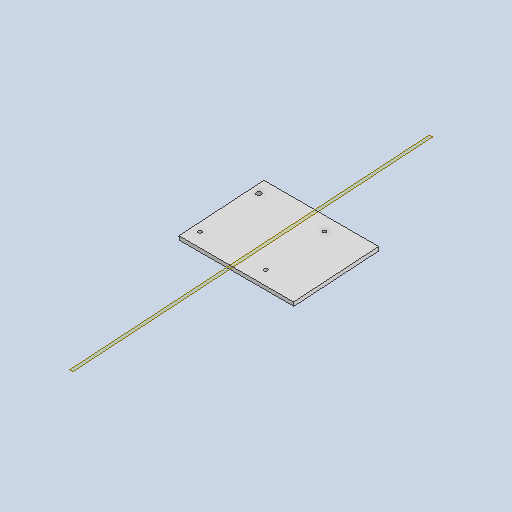
# Autodesk Inventor part: X axis carriage
Saved by Autodesk Inventor 2023.2 (Build 272271000, 271)
## iProperties
Created: 2023-05-09
Part Number: X axis carriage
Material: Generic
Document SubType Name: Modeling
Designer: dmargari
Density: 1 g/cm^3
Appearance: Default
Author: dmargari
Autodesk Inventor part; units mm, degrees
ref_plane "YZ Plane" through (0, 0, 0) normal (1, 0, 0) x (0, 1, 0)
ref_plane "XZ Plane" through (0, 0, 0) normal (0, 1, 0) x (-1, 0, 0)
ref_plane "XY Plane" through (0, 0, 0) normal (0, 0, 1) x (1, 0, 0)
ref_plane "Work Plane1" through (-11.5353, 732.2158, -211.5194) normal (-0.0000009, -0.9978756, -0.0651475) x (1, -0.0000009, -0.0000003)
sketch "Sketch2" plane through (-11.5353, 732.2158, -211.5194) normal (-0.0000009, -0.9978756, -0.0651475) x (1, -0.0000009, -0.0000003)
  line L0 (47.0205, 280.1712) -> (-77.9795, 280.1712)
  line L1 (-77.9795, 280.1712) -> (-77.9795, 150.1712)
  line L2 (-77.9795, 150.1712) -> (47.0205, 150.1712)
  line L3 (47.0205, 150.1712) -> (47.0205, 280.1712) construction
  line L4 (34.7205, 280.1712) -> (34.7205, 150.1712) construction
  line L5 (-65.6795, 280.1712) -> (-65.6795, 150.1712) construction
  circle A0 centre (34.7205, 260.1712) radius 2.55
  circle A1 centre (34.7205, 170.1712) radius 2.55
  circle A2 centre (-65.6795, 260.1712) radius 2.55
  circle A3 centre (-65.6795, 170.1712) radius 3.55
  line L6 (47.0205, 280.1712) -> (97.0205, 280.1712)
  line L7 (97.0205, 280.1712) -> (97.0205, 150.1712)
  line L8 (97.0205, 150.1712) -> (47.0205, 150.1712)
  point P0 (11.5359, 258.7721)
  point P1 (-138.0714, 537.573)
  point P2 (-211.9698, 678.1667)
  dimension "d15" = 125
  dimension "d16" = 130
  dimension "d17" = 12.3
  dimension "d18" = 12.3
  dimension "d19" = 5.1
  dimension "d20" = 5.1
  dimension "d21" = 5.1
  dimension "d22" = 7.1
  dimension "d23" = 50
  dimension "d24" = 20
  dimension "d25" = 20
  dimension "d26" = 20
  dimension "d27" = 20
  constraints: 18 end point, 9 point on line, 4 centre point, 4 perpendicular, 2 horizontal, 2 parallel, 1 collinear
  measures "d15" distance of L2.end L1.end
  measures "d16" distance of L1.end L0.end
  measures "d17" distance between parallel lines of L1 L5
  measures "d18" distance between parallel lines of L3 L4
  measures "d19" diameter of A0
  measures "d20" diameter of A1
  measures "d21" diameter of A2
  measures "d22" diameter of A3
  measures "d23" distance of L0.start L6.end
  measures "d24" distance from line of L2 A1.centre
  measures "d25" distance from line of L2 A3.centre
  measures "d26" distance from line of L0 A0.centre
  measures "d27" distance from line of L0 A2.centre
extrude "Extrusion2" add sketch "Sketch2" along normal blind 6
body "Solid2"
